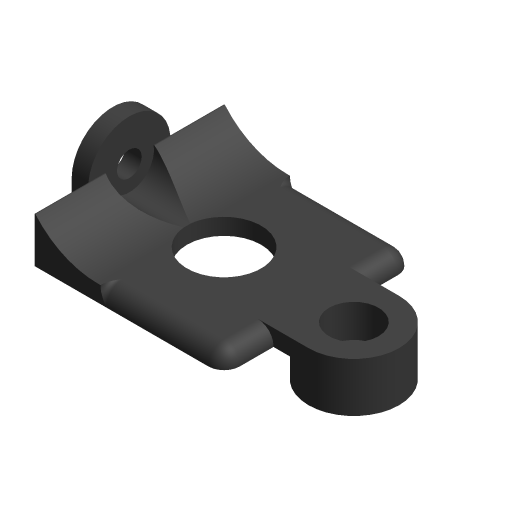
# Autodesk Inventor part: Camera retention
Saved by Autodesk Inventor 2024 (Build 280153000, 153)
## iProperties
Part Number: Camera retention
Material: Generic
Document SubType Name: Modeling
Designer: Jamie
Appearance: Default
Author: Jamie
Autodesk Inventor part; units mm, degrees
ref_plane "YZ Plane" through (0, 0, 0) normal (1, 0, 0) x (0, 1, 0)
ref_plane "XZ Plane" through (0, 0, 0) normal (0, 1, 0) x (-1, 0, 0)
ref_plane "XY Plane" through (0, 0, 0) normal (0, 0, 1) x (1, 0, 0)
sketch "Sketch27" plane through (0, 0, 0) normal (0, 1, 0) x (-1, 0, 0)
  circle A0 centre (0, 0) radius 4.5
  line L0 (11.5, 11.5) -> (-11.5, 11.5)
  line L1 (-11.5, -11.5) -> (11.5, -11.5)
  line L2 (11.5, -11.5) -> (11.5, 11.5)
  arc A1 (-15.75, 5.5) -> (-15.75, -5.5) centre (-15.75, 0) ccw
  circle A2 centre (-15.75, 0) radius 3
  line L3 (-15.75, 5.5) -> (-11.5, 5.5)
  line L4 (-15.75, -5.5) -> (-11.5, -5.5)
  line L5 (-11.5, 11.5) -> (-11.5, 5.5)
  line L6 (-11.5, -5.5) -> (-11.5, -11.5)
  dimension "d126" = 9
  dimension "d127" = 23
  dimension "d128" = 23
  dimension "d129" = 11.5
  dimension "d130" = 11.5
  dimension "d131" = 27.25
  dimension "d132" = 11
  dimension "d133" = 6
  dimension "d134" = 23
  dimension "d135" = 15.75
  constraints: 14 end point, 6 perpendicular, 3 centre point, 3 parallel, 2 coincident, 2 point on circle, 2 tangent, 1 horizontal
  measures "d126" diameter of A0
  measures "d127" distance of L1.end L1.start
  measures "d128" distance of L1.start L0.end
  measures "d129" distance from line of L1 point (0, 0)
  measures "d130" distance from line of L2 point (0, 0)
  measures "d131" distance from line of L2 A1.centre
  measures "d132" diameter of A1
  measures "d133" diameter of A2
  measures "d134" distance between parallel lines of L1 L0
  measures "d135" distance of point (0, 0) A1.centre
extrude "Extrusion22" add sketch "Sketch27" along normal blind 2
sketch "Sketch28" plane through (-11.5, 0, -11.5) normal (-1, 0, 0) x (0, 0, 1)
  circle A0 centre (11.5, 5) radius 1.5
  line L0 (0, 0) -> (23, 0) projected
  circle A1 centre (11.5, 5) radius 5
  line L1 (16.5, 5) -> (16.5, 0)
  line L2 (6.5, 5) -> (6.5, 0)
  point P0 (11.5, 0)
  point P1 (11.5, 0)
  dimension "d138" = 3
  dimension "d139" = 5
  dimension "d140" = 10
  constraints: 4 end point, 2 centre point, 2 point on circle, 2 point on line, 2 tangent, 1 coincident, 1 midpoint, 1 parallel, 1 perpendicular
  measures "d138" diameter of A0
  measures "d139" distance of point (11.5, 0) A0.centre
  measures "d140" diameter of A1
extrude "Extrusion23" add sketch "Sketch28" along normal blind 2
sketch "Sketch29" plane through (0, 0, 0) normal (0, -1, 0) x (1, 0, 0)
  circle A0 centre (15.75, 0) radius 3 projected
  circle A1 centre (15.75, 0) radius 5.5
  circle A2 centre (15.75, 0) radius 3
  line L0 (11.5, 5.5) -> (15.75, 5.5) projected
  line L1 (11.5, 5.5) -> (11.5, -5.5)
  point P0 (0, 0)
  point P1 (11.5, 3.4911)
  point P2 (11.5, -3.4911)
  dimension "d144" = 11
  dimension "d143" = 6
  constraints: 2 coincident, 2 end point, 1 centre point, 1 vertical, 2 other
  measures "d143" diameter of A2
extrude "Extrusion24" add sketch "Sketch29" along normal blind 2 contours A1 L1 picked at (11.9167, 0)
sketch "Sketch30" plane through (0, -2, 0) normal (0, -1, 0) x (1, 0, 0)
  circle A0 centre (15.75, 0) radius 1.5
  circle A1 centre (15.75, 0) radius 5.5
  line L0 (11.5, 5.5) -> (11.5, -5.5)
  point P0 (0, 0)
  point P1 (11.5, 3.4911)
  point P2 (11.5, -3.4911)
  dimension "d147" = 3
  constraints: 2 centre point, 2 coincident, 2 end point
  measures "d147" diameter of A0
extrude "Extrusion25" add sketch "Sketch30" along normal blind 2 contours A1 L0 picked at (12.4167, 0)
sketch "Sketch31" plane through (0, 2, 0) normal (0, 1, 0) x (1, 0, 0)
  line L0 (11.5, 11.5) -> (-11.5, 11.5) projected
  line L1 (-11.5, -11.5) -> (11.5, -11.5) projected
  line L2 (-11.5, 11.5) -> (-11.4, 11.5)
  line L3 (-11.4, 11.5) -> (-11.4, -11.5)
  line L4 (-11.4, -11.5) -> (-11.5, -11.5)
  line L5 (-11.5, -11.5) -> (-11.5, 11.5)
  point P0 (0, 0)
  dimension "d150" = 0.1
  constraints: 8 end point, 2 parallel, 1 horizontal, 1 perpendicular, 1 point on line
  measures "d150" distance of L3.end L4.end
extrude "Extrusion26" add sketch "Sketch31" along normal blind 3.5
fillet "Fillet10" radius 10 1 edges at (-11.4, 2, 0)
sketch "Sketch32" plane through (-11.5, 0, -11.5) normal (1, 0, 0) x (0, 0, -1)
  circle A0 centre (-11.5, 5) radius 3
  arc A1 (-6.5251, 5.5) -> (-16.4749, 5.5) centre (-11.5, 5) ccw projected
  point P0 (-11.5, 0)
  dimension "d154" = 6
  constraints: 1 centre point, 1 concentric
  measures "d154" diameter of A0
extrude "Extrusion27" cut sketch "Sketch32" along normal through all
sketch "Sketch33" plane through (11.5, 0, 11.5) normal (1, 0, 0) x (0, 0, -1)
  line L0 (17, 0) -> (23, 0) projected
  line L1 (23, 0) -> (20, 0)
  line L2 (20, 0) -> (20, 2.0077)
  line L3 (20, 2.0077) -> (21, 2.0077)
  line L4 (23, 0.0077) -> (23, 0)
  line L5 (0, 2) -> (9.0906, 2) projected
  line L6 (0, 0) -> (3.7675, 0)
  line L7 (3.7675, 0) -> (3.7675, 2)
  line L8 (3.7675, 2) -> (2, 2)
  line L9 (0, 0) -> (0, 0)
  arc A0 (23, 0.0077) -> (21, 2.0077) centre (21, 0.0077) ccw
  arc A1 (2, 2) -> (0, 0) centre (2, 0) ccw
  line L10 (20, 0) -> (23, 0)
  line L11 (23, 0) -> (23, 2)
  line L12 (23, 2) -> (20, 2)
  line L13 (20, 2) -> (20, 0)
  line L14 (3.7675, 0) -> (0, 0)
  line L15 (0, 0) -> (0, 2)
  line L16 (0, 2) -> (3.7675, 2)
  line L17 (3.7675, 2) -> (3.7675, 0)
  point P0 (11.5, 0)
  point P1 (21.1749, 2)
  point P2 (2, 2)
  dimension "d158" = 2
  constraints: 32 end point, 8 parallel, 4 horizontal, 4 perpendicular, 4 point on circle, 4 tangent, 2 centre point, 1 equal radius, 1 point on line
  measures "d158" radius of A0
extrude "Extrusion28" cut sketch "Sketch33" against normal blind 15 contours A0 L12 L11 | L5 A1 L15
fillet "Fillet13" radius 0.7 2 edges at (-3.5, 1.4142, 10.9142) (-3.5, 1.3586, -10.9747)
fillet "Fillet15" radius 1.9 5 edges at (11.5, 1.4142, 10.9142) (11.5, 2, 7.5) (11.5, 2, -7.5874) (11.5, 0.0038, -11.5) (11.5, 1.3586, -10.9747)
body "Solid3"
